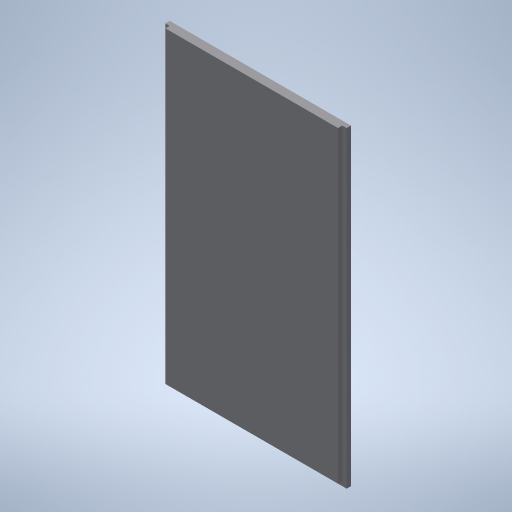
# Autodesk Inventor part: Tapa pared falsa
Saved by Autodesk Inventor 2023 (Build 270158000, 158)
## iProperties
Created: 2022-10-29
Part Number: Tapa pared falsa
Material: Generic
Document SubType Name: Modeling
Designer: Lenovo
Density: 1 g/cm^3
Appearance: Default
Author: Lenovo
Autodesk Inventor part; units mm, degrees
ref_plane "YZ Plane" through (0, 0, 0) normal (1, 0, 0) x (0, 1, 0)
ref_plane "XZ Plane" through (0, 0, 0) normal (0, 1, 0) x (-1, 0, 0)
ref_plane "XY Plane" through (0, 0, 0) normal (0, 0, 1) x (1, 0, 0)
sketch "Sketch1" plane through (0, 0, 0) normal (0, 0, 1) x (1, 0, 0)
  line L0 (0, 217) -> (126, 217)
  line L1 (126, 217) -> (126, 0)
  line L2 (126, 0) -> (0, 0)
  line L3 (0, 0) -> (0, 217)
  dimension "d0" = 126
  dimension "d1" = 217
  constraints: 8 end point, 2 parallel, 1 coincident, 1 horizontal, 1 perpendicular
  measures "d0" distance of L1.end L2.end
  measures "d1" distance of L0.end L1.end
extrude "Extrusion1" add sketch "Sketch1" along normal blind 3
sketch "Sketch2" plane through (0, 0, 3) normal (0, 0, 1) x (1, 0, 0)
  line L0 (0, 0) -> (126, 0) projected
  line L1 (126, 0) -> (126, 217) projected
  line L2 (126, 217) -> (0, 217) projected
  line L3 (0, 217) -> (0, 0) projected
  line L4 (3, 217) -> (123, 217)
  line L5 (123, 217) -> (123, 3)
  line L6 (123, 3) -> (3, 3)
  line L7 (3, 3) -> (3, 217)
  dimension "d4" = 3
  dimension "d5" = 3
  dimension "d6" = 3
  constraints: 8 end point, 2 parallel, 1 collinear, 1 horizontal, 1 perpendicular
  measures "d4" distance between parallel lines of L3 L7
  measures "d5" distance between parallel lines of L0 L6
  measures "d6" distance between parallel lines of L1 L5
extrude "Extrusion2" add sketch "Sketch2" along normal blind 3 contours L2 L5 L6 L7
body "Solid1"
